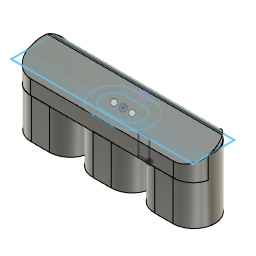
JD Fema holder v2 (Autodesk Fusion 360 design; units mm, degrees)
Autodesk Fusion 360 part; units mm, degrees
note: some values were not read from the file. Chosen so that the rebuilt part matches the saved one: which pieces of a blend or face edit are solid.
sketch "Sketch1" plane through (0, 0, 0) normal (0, 0, 1) x (1, 0, 0)
  line L0 (-2.5, 3.25) -> (2.5, 3.25)
  line L1 (2.5, -3.25) -> (-2.5, -3.25)
  arc A0 (2.5, -3.25) -> (2.5, 3.25) centre (2.5, 0) ccw
  arc A1 (-2.5, 3.25) -> (-2.5, -3.25) centre (-2.5, 0) ccw
  arc A2 (2.5, -5.75) -> (2.5, 5.75) centre (2.5, 0) ccw
  line L2 (-2.5, 5.75) -> (2.5, 5.75)
  arc A3 (-2.5, 5.75) -> (-2.5, -5.75) centre (-2.5, 0) ccw
  line L3 (2.5, -5.75) -> (-2.5, -5.75)
  dimension "d3" = 2.5
  dimension "d4" = 2.5
  dimension "d5" = -2.5
  constraint horizontal L0
  constraint parallel L0 L1
  measures "d3" distance of origin A0.centre
  measures "d4" distance of origin A1.centre
extrude "Extrude1" add sketch "Sketch1" along normal blind 2 contours L0 L1 A0 A1 | A2 L2 A3 L3 makes body 1
extrude "Extrude2" add sketch "Sketch1" against normal blind 15 bodies 1
sketch "Sketch2" plane through (0, 5.75, 0) normal (0, 1, 0) x (-1, 0, 0)
  line L0 (2.5, -15) -> (2.5, 2)
  line L1 (2.5, 2) -> (-2.5, 2)
  line L2 (-2.5, 2) -> (-2.5, -15)
  line L3 (-2.5, -15) -> (2.5, -15)
  line L4 (-1.5, -15) -> (1.5, -15)
  line L5 (1.5, -15) -> (1.5, -9.5)
  line L6 (1.5, -9.5) -> (-1.5, -9.5)
  line L7 (-1.5, -9.5) -> (-1.5, -15)
  dimension "d10" = 3
  dimension "d11" = 1.5
  dimension "d19" = 5.5
  constraint horizontal L4
  constraint vertical L5
  constraint horizontal L6
  constraint vertical L7
  constraint coincident L3 L4.start
  measures "d10" distance of L5.end L6.end
  measures "d11" horizontal distance of L6.end origin
  measures "d19" distance of L4 L6
extrude "Extrude3" add sketch "Sketch2" along normal blind 2.8 contours L3 L4 L5 L6 L7 bodies 1
chamfer "Chamfer1" distance 2.5 angle 45 1 edges at (0, 8.55, -15) on bodies 1
copy_body "CopyPasteBodies1" bodies 1 makes body 2
move_body "Move1" bodies 2 to x (1, 0, 0) y (0, 1, 0) z (0, 0, 1) at (17, 0, 0)
copy_body "CopyPasteBodies2" bodies 1 makes body 3
move_body "Move2" bodies 3 to x (1, 0, 0) y (0, 1, 0) z (0, 0, 1) at (-17, 0, 0)
sketch "Sketch3" plane through (0, 0, 2) normal (0, 0, 1) x (-1, 0, 0)
  arc A0 (2.5, -5.75) -> (2.5, 5.75) centre (2.5, 0) ccw
  line L0 (2.5, 5.75) -> (-2.5, 5.75)
  arc A1 (-2.5, 5.75) -> (-2.5, -5.75) centre (-2.5, 0) ccw
  line L1 (-2.5, -5.75) -> (2.5, -5.75)
  line L2 (25, -5.6312) -> (-25.0329, -5.6312)
  line L3 (-25.0329, -5.6312) -> (-25.0329, 5.8034)
  line L4 (-25.0329, 5.8034) -> (25, 5.8034)
  line L5 (25, 5.8034) -> (25, -5.6312)
  constraint horizontal L2
  constraint vertical L3
  constraint horizontal L4
  constraint vertical L5
extrude "Extrude4" add sketch "Sketch3" along normal blind -6 and the other way blind -2 contours A0 L0 A1 L2 | A0 L0 A1 L2 L3 L4 L5 bodies 1 2 3
chamfer "Chamfer2" distance 9 distance2 4 1 edges at (0.0165, -5.8034, 4) measured on face at (8.3553, -1.9918, 4) on bodies 1
fillet "Fillet1" radius 5.5 4 edges at (-25, -5.8034, -2) (-25, 5.6312, 0) (25.0329, -5.8034, -2) (25.0329, 5.6312, 0) on bodies 1
fillet "Fillet1" radius 2 1 edges at (0.0165, 5.6312, 4) on bodies 1
